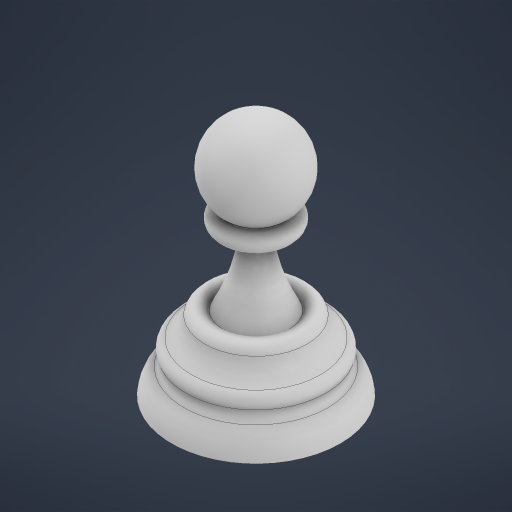
# Autodesk Inventor part: pěšec černý
Saved by Autodesk Inventor 2023 (Build 270158000, 158)
## iProperties
Created: 2023-04-20
Part Number: pěšec černý
Material: Generic
Document SubType Name: Modeling
Designer: 19LBoreckyP
Density: 1 g/cm^3
Appearance: Default
Author: 19LBoreckyP
Autodesk Inventor part; units mm, degrees
ref_plane "YZ Plane" through (0, 0, 0) normal (1, 0, 0) x (0, 1, 0)
ref_plane "XZ Plane" through (0, 0, 0) normal (0, 1, 0) x (-1, 0, 0)
ref_plane "XY Plane" through (0, 0, 0) normal (0, 0, 1) x (1, 0, 0)
sketch "Sketch1" plane through (0, 0, 0) normal (0, 0, 1) x (1, 0, 0)
  line L0 (17.5, 31.9391) -> (17.5, 33.9391)
  line L1 (23.1721, 29.9403) -> (22.2245, 29.9401)
  arc A0 (22.2245, 29.9401) -> (20.2449, 27.6586) centre (22.225, 27.9401) ccw
  arc A1 (35, 0.0037) -> (32.4419, 5.1885) centre (27.1551, -0.6434) ccw
  arc A2 (31.9987, 7.5695) -> (30.8857, 10.3325) centre (30.2268, 8.4614) ccw
  arc A3 (31.9987, 7.5695) -> (32.4419, 5.1885) centre (33.7851, 6.6703) ccw
  arc A4 (28.1124, 14.4594) -> (30.8857, 10.3325) centre (34.8187, 15.9709) ccw
  arc A5 (23.1721, 29.9403) -> (23.1909, 33.9402) centre (23.1717, 31.9403) ccw
  arc A6 (23.1909, 33.9402) -> (17.4895, 50) centre (17.5219, 40.9696) ccw
  arc A7 (103.989, 9.2063) -> (101.4308, 14.3911) centre (96.1441, 8.5592) ccw
  arc A8 (100.9877, 16.7722) -> (99.8747, 19.5351) centre (99.2158, 17.6641) ccw
  arc A9 (100.9877, 16.7722) -> (101.4308, 14.3911) centre (102.7741, 15.8729) ccw
  arc A10 (97.1014, 23.662) -> (99.8747, 19.5351) centre (103.8077, 25.1735) ccw
  arc A11 (97.1014, 23.662) -> (92.9704, 23.5655) centre (95.0456, 23.1987) ccw
  line L2 (103.989, 9.2026) -> (86.489, 9.2026)
  arc A12 (28.1124, 14.4594) -> (24.3692, 15.2585) centre (26.0566, 13.9961) ccw
  arc A13 (20.2449, 27.6586) -> (24.3692, 15.2585) centre (55.8089, 32.6015) ccw
  line L3 (17.4895, 50) -> (17.4968, 15.2585)
  line L4 (17.4968, 15.2585) -> (17.5, 0)
  line L5 (17.5, 0) -> (17.4895, 50)
  line L6 (17.5, 0) -> (35, 0.0037)
  point P0 (0, 0)
  dimension "d1" = 35
  dimension "d2" = 50
  dimension "d5" = 2
  dimension "d7" = 2
  dimension "d8" = 2
  dimension "d9" = 2
  constraints: 28 point on circle, 14 centre point, 14 end point, 8 tangent, 1 collinear, 1 horizontal, 1 perpendicular
  measures "d1" distance of point (0, 0) L6.end
  measures "d2" distance of L4.end L3.start
  measures "d5" distance of L0.start L0.end
  measures "d7" radius of A0
  measures "d8" radius of A3
  measures "d9" radius of A9
revolve "Revolution2" add sketch "Sketch1" angle 360 about axis through (17.5, 0, 0) along (-0.0002092, 1, 0)
body "Solid2"
